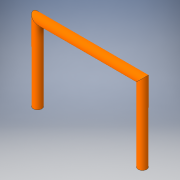
# Autodesk Inventor part: IED7_Sun_MouseTrap
Saved by Autodesk Inventor 2016 (Build 200138000, 138)
## iProperties
Created: 2017-11-09
Part Number: IED7_Sun_MouseTrap
Material: Generic
Document SubType Name: Modeling
Designer: sun01147
Density: 1 g/cm^3
Appearance: Default
Mass: 0.0646675 g
Surface Area: 1.88227 cm^2
Volume: 0.0646675 cm^3
Author: sun01147
Autodesk Inventor part; units mm, degrees
ref_plane "YZ Plane" through (0, 0, 0) normal (1, 0, 0) x (0, 1, 0)
ref_plane "XZ Plane" through (0, 0, 0) normal (0, 1, 0) x (-1, 0, 0)
ref_plane "XY Plane" through (0, 0, 0) normal (0, 0, 1) x (1, 0, 0)
sketch "Sketch1" plane through (0, 0, 0) normal (0, 0, 1) x (1, 0, 0)
  line L0 (0, 0) -> (0, 12.5222)
  line L1 (0, 12.5222) -> (17.145, 12.5222)
  line L2 (17.145, 12.5222) -> (17.145, 0)
  dimension "d1" = 12.5222
  dimension "d2" = 17.145
  dimension "d3" = 12.5222
  constraints: 6 end point, 2 vertical, 1 horizontal
  measures "d1" distance of L0.start L0.end
  measures "d2" distance of L0.end L1.end
  measures "d3" distance of L1.end L2.end
sketch "Sketch2" plane through (0, 0, 0) normal (0, 1, 0) x (-1, 0, 0)
  circle A0 centre (0, 0) radius 0.6985
  dimension "d4" = 1.397
  constraints: 1 centre point, 1 coincident
  measures "d4" diameter of A0
sweep "Sweep1" add profiles "Sketch2" path "Sketch1"
body "Solid1"
